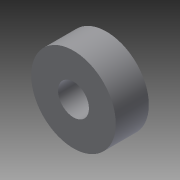
# Autodesk Inventor part: Small Bearing
Saved by Autodesk Inventor 2014 (Build 180170000, 170)
## iProperties
Created: 2015-02-07
Part Number: Small Bearing
Material: Generic
Document SubType Name: Modeling
Designer: Spooner
Density: 1 g/cm^3
Appearance: Default
Author: Spooner
Autodesk Inventor part; units mm, degrees
sketch "Sketch1" plane through (0, 0, 0) normal (0, 0, 1) x (1, 0, 0)
  circle A0 centre (0, 0) radius 13.0175
  circle A1 centre (0, 0) radius 4.7625
  dimension "d0" = 26.035
  dimension "d1" = 9.525
  constraints: 2 centre point, 2 coincident
  measures "d0" diameter of A0
  measures "d1" diameter of A1
extrude "Extrusion1" add sketch "Sketch1" along normal blind 10.16
ref_plane "Work Plane1" through (0, 0, 5.08) normal (0, 0, 1) x (1, 0, 0)
ref_plane "Work Plane2" through (0, 0, 0) normal (0, 1, 0) x (0, 0, 1)
ref_plane "Work Plane3" through (0, 0, 0) normal (1, 0, 0) x (0, 0, 1)
body "Solid1"
